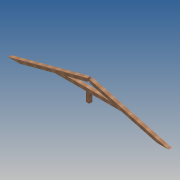
# Autodesk Inventor part: peak
Saved by Autodesk Inventor 2013 (Build 170138000, 138)
## iProperties
Created: 2013-08-10
Part Number: peak
Material: Wood (Birch)
Document SubType Name: Modeling
Designer: ddeboer
Mass: 24157.1 g
Surface Area: 20384.3 cm^2
Volume: 43922 cm^3
Density: 0.55 g/cm^3
Author: ddeboer
Autodesk Inventor part; units mm, degrees
ref_plane "YZ Plane" through (0, 0, 0) normal (1, 0, 0) x (0, 1, 0)
ref_plane "XZ Plane" through (0, 0, 0) normal (0, 1, 0) x (-1, 0, 0)
ref_plane "XY Plane" through (0, 0, 0) normal (0, 0, 1) x (1, 0, 0)
sketch "Sketch1" plane through (0, 0, 0) normal (0, 0, 1) x (1, 0, 0)
  line L0 (0, 0) -> (1828.8, 0) construction
  line L1 (0, 0) -> (1828.8, 490.0255)
  line L2 (1828.8, 0) -> (1828.8, 490.0255) construction
  line L3 (-319.438, 0) -> (1828.8, 575.6186)
  line L4 (1828.8, 490.0255) -> (1828.8, 575.6186)
  line L5 (0, 0) -> (-319.438, 0)
  line L6 (1828.8, 575.6186) -> (1873.25, 575.6186)
  line L7 (1873.25, 575.6186) -> (1873.25, 435.9186)
  line L8 (1873.25, 435.9186) -> (1828.8, 435.9186)
  line L9 (1828.8, 435.9186) -> (1828.8, 575.6186)
  line L10 (1851.025, 575.6186) -> (1851.025, 435.9186) construction
  line L11 (3702.05, 0) -> (1873.25, 490.0255)
  line L12 (4021.488, 0) -> (1873.25, 575.6186)
  line L13 (1873.25, 490.0255) -> (1873.25, 575.6186)
  line L14 (3702.05, 0) -> (4021.488, 0)
  line L15 (1784.35, 0) -> (1873.25, 0)
  line L16 (1873.25, 0) -> (1873.25, 254)
  line L17 (1873.25, 254) -> (1784.35, 254)
  line L18 (1784.35, 254) -> (1784.35, 0)
  line L19 (1828.8, 254) -> (1828.8, 0) construction
  line L20 (947.9409, 254) -> (2754.1091, 254)
  line L21 (2755.9432, 339.1017) -> (2755.9432, 342.9)
  line L22 (947.9409, 342.9) -> (947.9409, 339.5932)
  line L23 (960.2822, 342.9) -> (947.9409, 342.9)
  line L24 (2755.9432, 342.9) -> (2741.7678, 342.9)
  line L25 (2422.3298, 342.9) -> (1279.7202, 342.9)
  line L26 (947.9409, 254) -> (1279.7202, 342.9)
  line L27 (2422.3298, 342.9) -> (2754.1091, 254)
  dimension "d0" = 1828.8
  dimension "d1" = 15
  dimension "d2" = 139.7
  dimension "d3" = 44.45
  dimension "d4" = 254
  dimension "d5" = 88.9
  dimension "d6" = 88.9
  constraints: 56 end point, 8 parallel, 8 point on line, 5 perpendicular, 4 horizontal, 4 midpoint, 3 collinear, 3 symmetric about line
  measures "d0" distance of L0.start L0.end
  measures "d1" angle of L0 L1
  measures "d2" distance of L8.end L3.end
  measures "d3" distance of L3.end L6.end
  measures "d4" distance of L17.end L15.start
  measures "d5" distance of L15.start L15.end
  measures "d6" distance of L22.start L20.start
extrude "Extrusion1" add sketch "Sketch1" along normal blind 88.9 contours L5 L3 L4 L1 | L1 L25 L11 L20 L17 | L17 L16 L15 L18 | L11 L7 L12 L14
body "Solid1"
